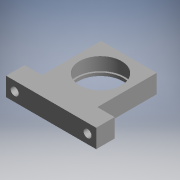
# Autodesk Inventor part: BSHKSA6904ZZ-40_h
Saved by Autodesk Inventor 2017.3 (Build 213256000, 256)
## iProperties
Part Number: BSHKSA6904ZZ-40_h
Material: Generic
Catalog Web Link: www.cadenas.de
Description: BSHKB, BSHK, BSHKA, BSHKSA, BSHFB, BSHF_housing-Bearings with Housings - with Positioning Groove - T-Shaped - Base Face Type
Vendor: MISUMI
Document SubType Name: Modeling
Designer: partserver
Manufacturer: MISUMI
Mass: 31.7655 g
Surface Area: 113.308 cm^2
Volume: 31.7655 cm^3
Density: 1 g/cm^3
Appearance: PSOLRGB-192-192-192
Category: PARTsolutions
Company: MISUMI
Title: BSHKSA6904ZZ-40
Author: Cadenas PARTsolutions
Comments: Bearings with Housings - with Positioning Groove - T-Shaped - Base Face Type
PSOL_IDENT_0: {$CADENAS_DATA\23d-libs\misumi\metric\12_bearing_holders\bshkb\housing_bshkb.prj},255 {VTYP=3D},{NB=
PSOL_IDENT_1: BSHKSA6904ZZ-40_h},{LINA=BSHKSA6904ZZ-40},{NN=BSHKB, BSHK, BSHKA, BSHKSA, BSHFB, BSHF_housing},{DATE=
PSOL_IDENT_2: 03.06.2021 05:36:04},{GEOMDATE=10.09.2019 05:28:41},{VERSION=},{LINEID=210},{WBVAR=TS,MATB,MATH,STH,
PSOL_IDENT_3: SEAL,HH,ALT1,ALT2,ALT3},{WBNUMERIC=HH}  {NB=BSHKSA6904ZZ-40_h},{LINA=BSHKSA6904ZZ-40},{KT=DUMMY},{PN=
PSOL_IDENT_4: BSHKSA6904ZZ-40},{TYPE=BSHKSA},{TS=HS},{TSALG= 'HS', 'Height h Selectable', 'HC', 'Height h Specifie
PSOL_IDENT_5: d' },{MATB=SST},{MATBALG= 'ST','Steel','SST','Stainless Steel' },{MATH=A2000},{MATH1= 'A2000','2017
PSOL_IDENT_6: Aluminum Alloy' },{STH=CA},{STH1=   'CA','Clear Anodizing'     },{ARR=304 Stainless Steel},{BN=6904}
PSOL_IDENT_7: ,{BN2=6904},{SEAL=ZZ},{SEALALG= 'ZZ', 'ZZ(Double Shielded)', 'VV', 'VV(Non-contact Rubber Seal)', 'D
PSOL_IDENT_8: D' , 'DD(Contact Rubber Seal)' },{HH=40},{HH1=40,50,60},{HH2=[30:80/1]},{DD=20},{D=37},{D3=39.800},{
PSOL_IDENT_9: BT=1.600},{DDHH=34},{B=9},{H=63},{HD1=23},{L=73},{L1=59},{L2=45},{L3=36.5},{T=15},{S=15},{DD1=6.5},{
PSOL_IDENT_10: TEMP1=2},{NR=},{HHALG=40,50,60},{ALT1=},{ALT1ALG= '', 'Bearing and Retaining Ring Assembled', 'NA'
PSOL_IDENT_11: , 'with NA (Bearing and Retaining Ring not Assembled)' },{ALT1PN=},{ALT2=},{ALT2ALG='', 'w/o Chamfer
PSOL_IDENT_12: ing', 'KCC', 'with KCC (C2 Chamfering)'},{ALT2PN=},{BNHALG=2},{ALT3=},{ALT3ALG= '','Not applicable'
PSOL_IDENT_13: },{ALT3PN=},{KKC=10}
NB: BSHKSA6904ZZ-40_h
NN: BSHKB, BSHK, BSHKA, BSHKSA, BSHFB, BSHF_housing
NT: Bearings with Housings - with Positioning Groove - T-Shaped - Base Face Type
NBSYN: $PN._h
LINA: BSHKSA6904ZZ-40
CATALOG: Misumi
PN: BSHKSA6904ZZ-40
TS: Height h Selectable
MATB: Stainless Steel
MATH: 2017 Aluminum Alloy
STH: Clear Anodizing
ARR: 304 Stainless Steel
BN: 6904
BN2: 6904
SEAL: ZZ(Double Shielded)
HH: 40
DD: 20
D: 37
D3: 39.8
BT: 1.6
DDHH: 34
B: 9
H: 63
HD1: 23
L: 73
L1: 59
L2: 45
L3: 36.5
T: 15
S: 15
DD1: 6.5
TEMP1: 2
ALT1: Bearing and Retaining Ring Assembled
ALT2: w/o Chamfering
ALT3: Not applicable
SUPPLIER: MISUMI
ARTICLENO: BSHKSA6904ZZ-40_h
BOMINFO: BSHKSA6904ZZ-40
CREATOR: CADENAS GmbH
Autodesk Inventor part; units mm, degrees
ref_plane "YZ Plane" through (0, 0, 0) normal (1, 0, 0) x (0, 1, 0)
ref_plane "XZ Plane" through (0, 0, 0) normal (0, 1, 0) x (-1, 0, 0)
ref_plane "XY Plane" through (0, 0, 0) normal (0, 0, 1) x (1, 0, 0)
sketch "Sketch_1" plane through (0, 0, 0) normal (0, 0, 1) x (1, 0, 0)
  line L0 (-36.5, -25) -> (-36.5, -40)
  line L1 (-36.5, -40) -> (36.5, -40)
  line L2 (36.5, -40) -> (36.5, -25)
  line L3 (36.5, -25) -> (22.5, -25)
  line L4 (22.5, -25) -> (22.5, 23)
  line L5 (22.5, 23) -> (-22.5, 23)
  line L6 (-22.5, 23) -> (-22.5, -25)
  line L7 (-22.5, -25) -> (-36.5, -25)
  constraints: 16 end point
extrude "Extrusion1" add sketch "Sketch_1" along normal mid plane 15
sketch "Sketch2" plane through (0, 0, 7.5) normal (0, 0, 1) x (1, 0, 0)
  point P0 (0, 0)
hole "Hole1" at (0, 0, 7.5) direction (0, 0, -1) diameter 34 depth 15 counterbore diameter 37 counterbore depth 13
sketch "Sketch3" plane through (-36.5, -40, 7.5) normal (0, -1, 0) x (1, 0, 0)
  point P0 (7, -7.5)
hole "Hole2" at (-29.5, -40, 0) direction (0, 1, 0) diameter 6.5 depth 15
sketch "Sketch4" plane through (-36.5, -40, 7.5) normal (0, -1, 0) x (1, 0, 0)
  point P0 (66, -7.5)
hole "Hole3" at (29.5, -40, 0) direction (0, 1, 0) diameter 6.5 depth 15
sketch "Sketch_7" plane through (0, 0, 3.5) normal (0, 0, 1) x (1, 0, 0)
  circle A0 centre (0, 0) radius 19.9
  constraints: 1 centre point
extrude "Extrusion2" cut sketch "Sketch_7" along normal blind 1.6
sketch "Sketch6" plane through (0, 0, 7.5) normal (0, 0, 1) x (1, 0, 0)
  point P0 (-29.5, -32.5)
hole "Hole4" at (-29.5, -32.5, 7.5) direction (0, 0, -1) diameter 3.25 depth 0.02
ref_plane "housing_to_dummy_XY" through (0, 0, 0) normal (1, 0, 0) x (0, 0, -1)
ref_plane "housing_to_dummy_YZ" through (0, 0, 0) normal (0, 0, -1) x (0, 1, 0)
ref_plane "housing_to_dummy_ZX" through (0, 0, 0) normal (0, 1, 0) x (1, 0, 0)
ref_plane "to_bearing_XY" through (0, 0, -5.5) normal (0, 0, 1) x (1, 0, 0)
ref_plane "to_bearing_YZ" through (0, 0, -5.5) normal (1, 0, 0) x (0, 1, 0)
ref_plane "to_bearing_ZX" through (0, 0, -5.5) normal (0, 1, 0) x (0, 0, 1)
ref_plane "to_rring_XY" through (0, 0, 3.5) normal (0, 0, -1) x (1, 0, 0)
ref_plane "to_rring_YZ" through (0, 0, 3.5) normal (1, 0, 0) x (0, -1, 0)
ref_plane "to_rring_ZX" through (0, 0, 3.5) normal (0, -1, 0) x (0, 0, -1)
body "Solid1"
